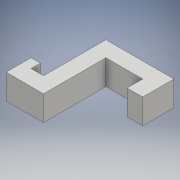
# Autodesk Inventor part: horizontal_clip
Saved by Autodesk Inventor 2018.3 (Build 223284000, 284)
## iProperties
Created: 2020-11-04
Part Number: horizontal_clip
Material: Generic
Document SubType Name: Modeling
Designer: chris
Density: 1 g/cm^3
Appearance: Default
Author: chris
Autodesk Inventor part; units mm, degrees
ref_plane "YZ Plane" through (0, 0, 0) normal (1, 0, 0) x (0, 1, 0)
ref_plane "XZ Plane" through (0, 0, 0) normal (0, 1, 0) x (-1, 0, 0)
ref_plane "XY Plane" through (0, 0, 0) normal (0, 0, 1) x (1, 0, 0)
sketch "Sketch1" plane through (0, 0, 0) normal (0, 0, 1) x (1, 0, 0)
  line L0 (-11.8, -20) -> (-23.8, -20)
  line L1 (-23.8, -20) -> (-23.8, -12)
  line L2 (-20.8, -15) -> (-16.8, -15)
  line L3 (-16.8, 5) -> (-16.8, -15)
  line L4 (-11.8, -20) -> (-11.8, 0)
  line L5 (-11.8, 0) -> (0, 0)
  line L6 (0, 0) -> (0, -5)
  line L7 (0, -5) -> (5, -5)
  line L8 (5, -5) -> (5, 5)
  line L9 (5, 5) -> (-16.8, 5)
  line L10 (-23.8, -12) -> (-20.8, -12)
  line L11 (-20.8, -12) -> (-20.8, -15)
  constraints: 24 end point, 5 vertical, 3 horizontal, 3 perpendicular
extrude "Extrusion1" add sketch "Sketch1" along normal blind 8
body "Solid1"
